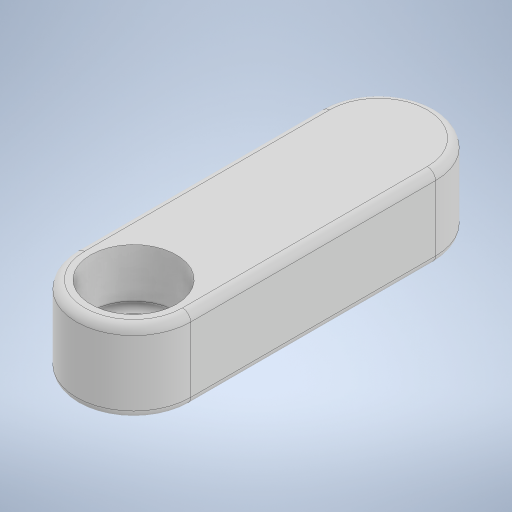
# Autodesk Inventor part: v2batterylock
Saved by Autodesk Inventor 2024.2 (Build 282272000, 272)
## iProperties
Created: 2024-01-13
Part Number: v2batterylock
Material: Generic
Document SubType Name: Modeling
Designer: Eric
Density: 1 g/cm^3
Appearance: Default
Author: Eric
Autodesk Inventor part; units mm, degrees
ref_plane "YZ Plane" through (0, 0, 0) normal (1, 0, 0) x (0, 1, 0)
ref_plane "XZ Plane" through (0, 0, 0) normal (0, 1, 0) x (-1, 0, 0)
ref_plane "XY Plane" through (0, 0, 0) normal (0, 0, 1) x (1, 0, 0)
sketch "Sketch1" plane through (0, 0, 0) normal (0, 1, 0) x (-1, 0, 0)
  line L0 (0, 0) -> (0, -15) construction
  line L1 (-3.5, 0) -> (-3.5, -15)
  line L2 (3.5, -15) -> (3.5, 0)
  arc A0 (3.5, 0) -> (-3.5, 0) centre (0, 0) ccw
  arc A1 (-3.5, -15) -> (3.5, -15) centre (0, -15) ccw
  circle A2 centre (0, 0) radius 1.7
  point P0 (0, -7.5)
  dimension "d0" = 7
  dimension "d1" = 15
  dimension "d2" = 3.4
  constraints: 8 end point, 4 point on circle, 4 tangent, 3 centre point, 1 coincident, 1 midpoint, 1 parallel, 1 vertical
  measures "d0" distance between parallel lines of L2 L1
  measures "d1" distance of L0.end L0.start
  measures "d2" diameter of A2
extrude "Extrusion1" add sketch "Sketch1" along normal blind 5
sketch "Sketch2" plane through (0, 5, 0) normal (0, 1, 0) x (1, 0, 0)
  circle A0 centre (0, 0) radius 2.625
  dimension "d5" = 5.25
  constraints: 1 centre point, 1 coincident
  measures "d5" diameter of A0
extrude "Extrusion2" cut sketch "Sketch2" against normal blind 3
fillet "Fillet1" radius 0.5 8 edges at (0, 0, -18.5) (-3.5, 0, -7.5) (0, 0, 3.5) (3.5, 0, -7.5) (0, 5, -18.5) (-3.5, 5, -7.5) (0, 5, 3.5) (3.5, 5, -7.5)
body "Solid1"
